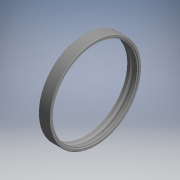
# Autodesk Inventor part: W 61705-2RZ_PART2
Saved by Autodesk Inventor 2017.3 (Build 213256000, 256)
## iProperties
Part Number: W 61705-2RZ_PART2
Material: Generic
Catalog Web Link: www.cadenas.de
Description: -Deep groove ball bearings
Vendor: SKF
Document SubType Name: Modeling
Designer: partserver
Manufacturer: SKF
Mass: 0.438086 g
Surface Area: 10.0178 cm^2
Volume: 0.438086 cm^3
Density: 1 g/cm^3
Appearance: PSOLRGB-175-175-175
Category: PARTsolutions
Company: SKF
Title: W 61705-2RZ_PART2
Author: Cadenas PARTsolutions
Comments: Deep groove ball bearings
PSOL_IDENT_0: {$CADENAS_DATA\23d-libs\skf\bearings_units_and_housings\ball_bearings\deep_groove_ball_bearings\bb1_
PSOL_IDENT_1: 001_101.prj},201 {VTYP=3D},{NB=W 61705-2RZ_PART2},{LINA=W 61705-2RZ_PART2},{NN=BB1_001_101_PART2},{N
PSOL_IDENT_2: OPRJ=TRUE},{DATE=19.12.2019 14:34:47},{GEOMDATE=18.12.2019 13:53:11},{VERSION=},{LINEID=17800},{WBVA
PSOL_IDENT_3: R=},{WBNUMERIC=}  {NB=W 61705-2RZ_PART2},{LINA=W 61705-2RZ_PART2},{KT=DUMMY},{PRODUCTID=},{DESIGNATI
PSOL_IDENT_4: ON=W 61705-2RZ},{DD=25.000},{D=32.000},{B=4.000},{C=0.000},{DD1=27.27},{DD2=0.00},{D1=0.00},{D2=30.2
PSOL_IDENT_5: 9},{D3=0.000},{D4=0.000},{HH=MIN},{BB=0.000},{FF=0.00},{R0MAX=MIN},{R0=MIN},{R12=0.20},{PITCH=28.50}
PSOL_IDENT_6: ,{DW=1.588},{DDAMIN=26.500},{DDAMAX=27.000},{DDBMIN=MIN},{DDBMAX=MIN},{DBMIN=MIN},{DAMAX=30.500},{BB
PSOL_IDENT_7: AMIN=MIN},{CAMAX=MIN},{RAMAX=0.200},{LOAD1=0.618},{LOAD2=0.465},{LOAD3=0.020},{SPEED1=43000},{SPEED2=
PSOL_IDENT_8: 20000},{KR=0.015},{F0=8.800},{Z=21},{II=1},{MASS=0.007},{BEARING=W 61705-2RZ},{RING=},{HELP=1.218},{
PSOL_IDENT_9: HELP2=0.855},{DD1ALG=13.635},{YALG=13.635},{PITCH1=28.500},{DW1=1.588},{YALG1=14.782},{HALG1=1.218},
PSOL_IDENT_10: {SH=13.635},{CU=0.482},{DESIGN=dgbb2rs},{HALG=1.135},{B1=0},{SHIELDHELP=2}
NB: W 61705-2RZ_PART2
NT: Deep groove ball bearings
NBSYN: $DESIGNATION._PART2
LINA: W 61705-2RZ_PART2
CATALOG: SKF
SUPPLIER: SKF
ARTICLENO: W 61705-2RZ_PART2
BOMINFO: W 61705-2RZ_PART2
CREATOR: CADENAS GmbH
Autodesk Inventor part; units mm, degrees
ref_plane "YZ Plane" through (0, 0, 0) normal (1, 0, 0) x (0, 1, 0)
ref_plane "XZ Plane" through (0, 0, 0) normal (0, 1, 0) x (-1, 0, 0)
ref_plane "XY Plane" through (0, 0, 0) normal (0, 0, 1) x (1, 0, 0)
sketch "Sketch_9" plane through (0, 0, 0) normal (0, 0, 1) x (1, 0, 0)
  line L0 (50, 0) -> (-50, 0)
  line L1 (0, 15.8) -> (0, 15.145)
  line L2 (0, 15.145) -> (0.1, 15.145)
  arc A0 (0.3, 14.945) -> (0.1, 15.145) centre (0.1, 14.945) ccw
  line L3 (0.3, 14.945) -> (0.3, 14.745)
  line L4 (0.3, 14.745) -> (1.3792, 14.745)
  arc A1 (2.6208, 14.745) -> (1.3792, 14.745) centre (2, 14.25) ccw
  line L5 (2.6208, 14.745) -> (3.7, 14.745)
  line L6 (3.7, 14.745) -> (3.7, 14.945)
  arc A2 (3.9, 15.145) -> (3.7, 14.945) centre (3.9, 14.945) ccw
  line L7 (3.9, 15.145) -> (4, 15.145)
  line L8 (4, 15.145) -> (4, 15.8)
  arc A3 (4, 15.8) -> (3.8, 16) centre (3.8, 15.8) ccw
  line L9 (3.8, 16) -> (0.2, 16)
  arc A4 (0.2, 16) -> (0, 15.8) centre (0.2, 15.8) ccw
  constraints: 20 end point, 10 point on circle, 5 centre point
revolve "Revolution1" add sketch "Sketch_9" angle 360 about axis through (50, 0, 0) along (1, 0, 0)
body "Solid1"
